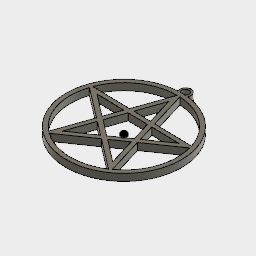
星型挂件 v0 (Autodesk Fusion 360 design; units mm, degrees)
Autodesk Fusion 360 part; units mm, degrees
sketch "草图1" plane through (0, 0, 0) normal (0, 1, 0) x (1, 0, 0)
sketch "草图2" plane through (0, 0, 0) normal (0, 1, 0) x (1, 0, 0)
  circle A0 centre (0, 0) radius 40.6099
  line L0 (-0.1456, 37.6096) -> (-8.8372, 12.7481)
  line L1 (0.6847, 30.8941) -> (-5.6836, 12.6782)
  line L2 (-35.1678, 13.3317) -> (-8.8372, 12.7481)
  line L3 (-29.1705, 10.198) -> (-9.8782, 9.7704)
  line L4 (-29.1705, 10.198) -> (-13.814, -1.4876)
  line L5 (-9.8782, 9.7704) -> (-13.814, -1.4876)
  line L6 (-14.855, -4.4653) -> (-23.5466, -29.3268)
  line L7 (-6.7246, 9.7005) -> (-11.3038, -3.3978)
  line L8 (-12.3448, -6.3755) -> (-18.713, -24.5914)
  line L9 (-35.8139, 11.4835) -> (-14.855, -4.4653)
  line L10 (-12.3448, -6.3755) -> (-2.8539, -13.5976)
  line L11 (-0.3437, -15.5078) -> (20.6152, -31.4566)
  line L12 (-2.8539, -13.5976) -> (-18.713, -24.5914)
  line L13 (-11.3038, -3.3978) -> (-0.2615, -11.8005)
  line L14 (2.2487, -13.7107) -> (17.6052, -25.3963)
  line L15 (-0.3437, -15.5078) -> (-21.9886, -30.5124)
  line L16 (36.2875, 9.8856) -> (14.6426, -5.119)
  line L17 (12.0502, -6.9162) -> (2.2487, -13.7107)
  line L18 (17.6052, -25.3963) -> (12.0502, -6.9162)
  line L19 (29.5936, 8.8956) -> (13.7345, -2.0982)
  line L20 (11.1421, -3.8953) -> (-0.2615, -11.8005)
  line L21 (22.2242, -30.3412) -> (14.6426, -5.119)
  line L22 (-6.7246, 9.7005) -> (7.1477, 9.3931)
  line L23 (10.3014, 9.3232) -> (29.5936, 8.8956)
  line L24 (11.1421, -3.8953) -> (7.1477, 9.3931)
  line L25 (6.2397, 12.4139) -> (0.6847, 30.8941)
  line L26 (13.7345, -2.0982) -> (10.3014, 9.3232)
  line L27 (9.3933, 12.344) -> (1.8117, 37.5662)
  line L28 (-5.6836, 12.6782) -> (6.2397, 12.4139)
  line L29 (9.3933, 12.344) -> (35.7239, 11.7605)
  arc A1 (-0.1456, 37.6096) -> (-35.1678, 13.3317) centre (0, 0) ccw
  arc A2 (35.7239, 11.7605) -> (1.8117, 37.5662) centre (0, 0) ccw
  arc A3 (22.2242, -30.3412) -> (36.2875, 9.8856) centre (0, 0) ccw
  arc A4 (-35.8139, 11.4835) -> (-23.5466, -29.3268) centre (0, 0) ccw
  arc A5 (-21.9886, -30.5124) -> (20.6152, -31.4566) centre (0, 0) ccw
  point P0 (0.6847, 30.8941)
  point P1 (-18.713, -24.5914)
  point P2 (-29.1705, 10.198)
  point P3 (29.5936, 8.8956)
  point P4 (17.6052, -25.3963)
sketch "草图3" plane through (0, 0, 0) normal (0, 1, 0) x (1, 0, 0)
sketch "草图4" plane through (0, 0, 0) normal (0, 1, 0) x (1, 0, 0)
sketch "草图5" plane through (0, 0, 0) normal (0, 1, 0) x (1, 0, 0)
sketch "草图6" plane through (0, 0, 0) normal (0, 1, 0) x (1, 0, 0)
extrude "拉伸1" add sketch "草图2" along normal blind 5 makes body 1
sketch "草图7" plane through (0, 0, 0) normal (0, 1, 0) x (1, 0, 0)
  circle A0 centre (-61, 0) radius 2.5
  circle A1 centre (-61, 0) radius 4
extrude "拉伸2" add sketch "草图7" along normal blind 5 separate body makes body 2
move_body "移动1" bodies 2 to x (1, 0, 0) y (0, 1, 0) z (0, 0, 1) at (61.9455, 0, -42.3352)
combine "合并1" operation add target body 2 tool bodies 1
